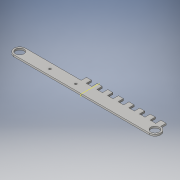
# Autodesk Inventor part: Sidewall
Saved by Autodesk Inventor 2016 (Build 200138000, 138)
## iProperties
Created: 2016-02-15
Part Number: Sidewall
Material: Generic
Document SubType Name: Modeling
Designer: Michael
Density: 1 g/cm^3
Appearance: Default
Author: Michael
Autodesk Inventor part; units mm, degrees
ref_plane "YZ Plane" through (0, 0, 0) normal (1, 0, 0) x (0, 1, 0)
ref_plane "XZ Plane" through (0, 0, 0) normal (0, 1, 0) x (-1, 0, 0)
ref_plane "XY Plane" through (0, 0, 0) normal (0, 0, 1) x (1, 0, 0)
sketch "Sketch1" plane through (0, 0, 0) normal (0, 1, 0) x (-1, 0, 0)
  line L0 (69, 5.4) -> (-69, 5.4)
  line L1 (-69, 5.4) -> (-69, -5.4)
  line L2 (-69, -5.4) -> (69, -5.4)
  line L3 (69, -5.4) -> (69, 5.4)
  line L4 (69, 5.4) -> (-69, -5.4) construction
  line L5 (-69, 5.4) -> (69, -5.4) construction
  circle A0 centre (35.2, 0) radius 1
  circle A1 centre (10.8, 0) radius 1
  circle A2 centre (63.6, 0) radius 4
  point P0 (0, 0)
  dimension "d0" = 138
  dimension "d1" = 10.8
  dimension "d2" = 2
  dimension "d3" = 2
  dimension "d4" = 33.8
  dimension "d5" = 58.2
  dimension "d6" = 8
  dimension "d7" = 5.4
  constraints: 12 end point, 3 centre point, 2 midpoint, 2 parallel, 1 horizontal, 1 perpendicular
  measures "d0" distance of L2.end L1.end
  measures "d1" distance of L0.end L1.end
  measures "d2" diameter of A0
  measures "d3" diameter of A1
  measures "d4" distance from line of L3 A0.centre
  measures "d5" distance from line of L3 A1.centre
  measures "d6" diameter of A2
  measures "d7" distance from line of L3 A2.centre
extrude "Extrusion1" add sketch "Sketch1" along normal blind 1.6
full round fillet "Fillet1" first side at (-23, 1.0667, 5.4) centre faces at (-69, 0.5333, -1.8) second side at (23, 1.0667, -5.4)
mirror "Mirror1" about plane through (0, 0, 0) normal (1, 0, 0) of "Fillet1"
sketch "Sketch2" plane through (0, 1.6, 0) normal (0, 1, 0) x (1, 0, 0)
  circle A0 centre (63.6, 0) radius 4
  arc A1 (63.6, -5.4) -> (63.6, 5.4) centre (63.6, 0) ccw projected
  point P0 (0, 0)
  dimension "d10" = 8
  dimension "d11" = 0
  constraints: 1 centre point
  measures "d10" diameter of A0
  measures "d11" distance of A1.centre A0.centre
extrude "Extrusion2" cut sketch "Sketch2" against normal blind 1.6
sketch "Sketch3" plane through (0, 1.6, 0) normal (0, 1, 0) x (1, 0, 0)
  line L0 (63.6, 5.4) -> (-63.6, 5.4) projected
  circle A0 centre (63.6, 0) radius 4 projected
  circle A1 centre (-63.6, 0) radius 4 projected
  circle A2 centre (-10.8, 0) radius 1 projected
  circle A3 centre (-35.2, 0) radius 1 projected
  arc A4 (63.6, -5.4) -> (63.6, 5.4) centre (63.6, 0) ccw projected
  line L1 (63.6, 5.4) -> (-63.6, 5.4) projected
  arc A5 (-63.6, 5.4) -> (-63.6, -5.4) centre (-63.6, 0) ccw projected
  line L2 (-63.6, -5.4) -> (63.6, -5.4) projected
  line L3 (63.6, 5.4) -> (58.8, 5.4)
  line L4 (58.8, 5.4) -> (58.8, 10.4)
  line L5 (58.8, 10.4) -> (63.6, 10.4)
  line L6 (63.6, 10.4) -> (63.6, 5.4)
  point P0 (0, 0)
  dimension "d16" = 4.8
  dimension "d17" = 5
  constraints: 8 end point, 2 parallel, 1 perpendicular, 1 point on line
  measures "d16" distance of L1.start L3.end
  measures "d17" distance of L3.end L4.end
extrude "Extrusion3" add sketch "Sketch3" against normal blind 1.6 contours L0 L4 L5 L6
pattern_linear "Rectangular Pattern1" count 8 spacing 10 along (-1, 0, 0) of "Extrusion3"
ref_plane "Work Plane1" through (0, 0, 0) normal (1, 0, 0) x (0, 1, 0)
body "Solid1"
